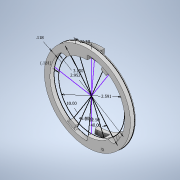
# Autodesk Inventor part: lock
Saved by Autodesk Inventor 2020 (Build 240168000, 168)
## iProperties
Created: 2022-01-17
Part Number: lock
Material: Generic
Document SubType Name: Modeling
Designer: gamma
Density: 1 g/cm^3
Appearance: Default
Author: gamma
Autodesk Inventor part; units mm, degrees
ref_plane "YZ Plane" through (0, 0, 0) normal (1, 0, 0) x (0, 1, 0)
ref_plane "XZ Plane" through (0, 0, 0) normal (0, 1, 0) x (-1, 0, 0)
ref_plane "XY Plane" through (0, 0, 0) normal (0, 0, 1) x (1, 0, 0)
sketch "Sketch1" plane through (0, 0, 0) normal (0, 0, 1) x (1, 0, 0)
  circle A0 centre (0, 0) radius 32.9
  circle A1 centre (0, 0) radius 37.4904
  circle A2 centre (0, 0) radius 40.005
  line L0 (0, 0) -> (-36.9208, 6.5101)
  line L1 (0, 40.005) -> (0, -40.005)
  line L2 (0, 0) -> (-3.4867, -39.8528)
  line L3 (0, 0) -> (3.4867, 39.8528)
  line L4 (0, 0) -> (25.7147, -30.6456)
  line L5 (0, 0) -> (15.3093, -36.9598)
  line L6 (0, 0) -> (-25.7147, 30.6456)
  line L7 (0, 0) -> (-15.3093, 36.9598)
  circle A3 centre (15.3093, -36.9598) radius 1.1653
  line L8 (0, 0) -> (-15.3093, -36.9598)
  line L9 (0, 0) -> (15.3093, 36.9598)
  line L10 (0, 0) -> (-21.4947, -33.7399)
  line L11 (0, 0) -> (21.4947, 33.7399)
  circle A4 centre (0, 0) radius 43.005
  point P0 (-24.0984, 28.7193)
  point P1 (-21.1477, 25.2029)
  point P2 (0, 32.9)
  point P3 (0, 37.4904)
  point P4 (24.0984, -28.7193)
  point P5 (21.1477, -25.2029)
  point P6 (0, -32.9)
  point P7 (0, -37.4904)
  point P8 (14.2262, -37.39)
  point P9 (16.3793, -36.4982)
  point P10 (-2.8674, -32.7748)
  point P11 (-3.2675, -37.3477)
  point P12 (2.8674, 32.7748)
  point P13 (3.2675, 37.3477)
  point P14 (14.347, -34.6366)
  point P15 (12.5903, -30.3956)
  point P16 (-14.347, 34.6366)
  point P17 (-12.5903, 30.3956)
  point P18 (17.6772, 27.7476)
  point P19 (20.1436, 31.6191)
  point P20 (14.347, 34.6366)
  point P21 (12.5903, 30.3956)
  point P22 (-17.6772, -27.7476)
  point P23 (-20.1436, -31.6191)
  point P24 (-14.347, -34.6366)
  point P25 (-12.5903, -30.3956)
  dimension "d1" = 74.9808
  dimension "d8" = 80.01
  dimension "d0" = 65.8
  dimension "d2" = 4.5904
  dimension "d12" = 5
  dimension "d13" = 40
  dimension "d14" = 22.5
  dimension "d15" = 22.5
  dimension "d23" = 45
  dimension "d24" = 10
  dimension "d31" = 3
  constraints: 24 end point, 5 coincident, 3 centre point, 2 point on line, 1 vertical, 17 other
  measures "d0" diameter of A0
  measures "d12" angle of L1 L2
  measures "d13" angle of L1 L4
  measures "d14" angle of L1 L5
  measures "d15" angle of L1 L7
  measures "d23" angle of L8 L5
  measures "d24" angle of L10 L8
extrude "Extrusion1" add sketch "Sketch1" along normal blind 4 contours L4 A1 L5 A0 | L11 A2 L4 A1 | A1 L9 A2 L11 | L5 A1 L1 A0 | L4 A2 A3 L5 A1 | A1 L3 A2 L9 | A0 L7 A1 L1 | L6 A1 L7 A0 | L5 A3 A2 L1 A1 | A1 L1 A2 L3 | A1 L10 A2 L6 | A1 L7 A2 L1 | L1 A2 L2 A1 | L2 A2 L8 A1 | L6 A2 L7 A1 | L8 A2 L10 A1 | A4
extrude "Extrusion2" add sketch "Sketch1" against normal blind 10 contours L4 A1 L5 A0 | L5 A1 L1 A0 | A0 L1 A1 L3 | A0 L7 A1 L1 | L1 A1 L2 A0 | L6 A1 L7 A0
extrude "Extrusion3" cut sketch "Sketch1" against normal blind 6.18 contours L5 A1 L1 A0 | A0 L7 A1 L1
extrude "Extrusion4" cut sketch "Sketch1" against normal blind 5.9 contours A0 L1 A1 L3 | L1 A1 L2 A0
fillet "Fillet1" radius 1.016 4 edges at (0, 35.1952, -5.9) (3.0675, 35.0613, -5.9) (0, -35.1952, -5.9) (-3.0675, -35.0613, -5.9)
extrude "Extrusion5" add sketch "Sketch1" along normal blind 3 contours A0 L9 A1 L11 | L8 A1 L10 A0
fillet "Fillet2" radius 5.08 2 edges at (-24.0984, 28.7193, 2) (24.0984, -28.7193, 2)
fillet "Fillet3" radius 5.08 2 edges at (-22.623, 26.9611, 0) (22.623, -26.9611, 0)
fillet "Fillet4" radius 1.27 2 edges at (13.4686, -32.5161, -6.18) (-13.4686, 32.5161, -6.18)
fillet "Fillet5" radius 1.27 6 edges at (0, -37.4904, 2) (0, 37.4904, 2) (14.347, 34.6366, 1.5) (20.1436, 31.6191, 1.5) (-14.347, -34.6366, 1.5) (-20.1436, -31.6191, 1.5)
extrude "Extrusion6" add sketch "Sketch1" against normal blind 1
body "Solid1"
